centerHolderTop_v2 (Autodesk Fusion 360 design; units mm, degrees)
Autodesk Fusion 360 part; units mm, degrees
note: some values were not read from the file. Set by a fixed rule: which face or edge a step refers to.
sketch "Sketch1" plane through (0, 0, 0) normal (0, 0, 1) x (1, 0, 0)
  circle A0 centre (0, 0) radius 6.35
  circle A1 centre (0, 0) radius 9.525
  dimension "d1" = 12.7
  dimension "d24" = 19.05
  constraint coincident A0.centre A1.centre
  measures "d1" diameter of A0
  measures "d24" diameter of A1
extrude "Extrude1" add sketch "Sketch1" along normal blind 12.7 contours A0
ref_plane "WorkPlane1" through (0, -6.35, 16.0163) normal (0, -1, 0) x (-1, 0, 0)
sketch "Sketch2" plane through (0, -6.35, 16.0163) normal (0, -1, 0) x (1, 0, 0)
  line L0 (6.35, -3.3163) -> (-6.35, -3.3163)
  line L1 (6.35, -16.0163) -> (-6.35, -16.0163)
  point P0 (0, -3.3163)
  constraint midpoint L0 P0
ref_plane "WorkPlane2" through (0, 0, 9.525) normal (0, 0, 1) x (1, 0, 0)
sketch "Sketch4" plane through (0, 0, 9.525) normal (0, 0, 1) x (1, 0, 0)
  circle A0 centre (0, 0) radius 6.35
  line L0 (0, 0) -> (0, -6.35) construction
  line L1 (0, 0) -> (5.4993, 3.175) construction
  line L2 (0, 0) -> (-5.4993, 3.175) construction
  dimension "d22" = 360
  constraint coincident A0.centre L0.start
  constraint coincident A0 L0.end
  constraint vertical L0
hole "Hole1" at (0, -6.35, 12.7) direction (0, 1, 0) diameter 6.35 depth 6.35 tip angle 180
pattern_circular "C-Pattern1" count 3 over 360 about axis through (0, 0, 0) along (0, 0, 1) of "Hole1"
extrude "Extrude2" cut sketch "Sketch4" against normal blind 0.127 from surface at 3.175
hole "Hole2" at (0, 0, 0) direction (0, 0, 1) diameter 3.2639 depth 12.573 tip angle 180
extrude "Extrude3" add sketch "Sketch1" along normal blind 3.175
equation "d5 = d1 / 2"
